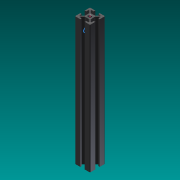
# Autodesk Inventor part: NFS5-2020-170-TPW
Saved by Autodesk Inventor 2015 (Build 190159000, 159)
## iProperties
Category: PARTsolutions
Company: MISUMI
Created: 2016-02-17
Part Number: NFS5-2020-170-TPW
Catalog Web Link: www.cadenas.de
Description: NFS5-2020, NFSB5-2020, HFS5-2020, HFSB5-2020, CAF5-2020, HFSY5-2020, NFSF5-2020, HFSF5-2020, HFSFB5-2020, NFST5-2020, HFST5-2020, HFSTB5-2020, HFSH5-2020, HFSC5-2020-HFS5 Series Aluminum Extrusions 20 Square -1 Slot-
Vendor: MISUMI
Document SubType Name: Modeling
Designer: psAdmin
Manufacturer: MISUMI
Mass: 30.8251 g
Surface Area: 299.433 cm^2
Volume: 30.8251 cm^3
Density: 1 g/cm^3
Material: 一般
Appearance: PSOLRGB-175-175-175
PSOL_IDENT_0: {$CADENAS_DATA\23d-libs\misumi\metric\38_al_extrusions_blackets\5\hfs5_2020.prj},577 {VTYP=3D},{NB=N
PSOL_IDENT_1: FS5-2020-170-TPW},{LINA=NFS5-2020-170-TPW},{NN=NFS5-2020, NFSB5-2020, HFS5-2020, HFSB5-2020, CAF5-20
PSOL_IDENT_2: 20, HFSY5-2020, NFSF5-2020, HFSF5-2020, HFSFB5-2020, NFST5-2020, HFST5-2020, HFSTB5-2020, HFSH5-2020
PSOL_IDENT_3: , HFSC5-2020},{DATE=17.07.2015 10:47:07},{GEOMDATE=28.10.2014 00:00:00},{VERSION=},{LINEID=10},{LINE
PSOL_IDENT_4: SUBID=-1},{WBVAR=L,ALT1,ALT2,ALT4,ALT5,CP5,DL5,DR5,ALT6,ALT9,ALT10,ALT11,HP6,NHL6,DL6,NHR6,DR6,ALT7,
PSOL_IDENT_5: ALT8,NH9,AH,BH,CH,DH,EH,NH10,AV,BV,CV,DV,EV,NH11,AP,BP,CP,DP,EP,ALT12,ALT13,Z,NH12,XA,XB,XC,XD,XE,NH
PSOL_IDENT_6: 13,YA,YB,YC,YD,YE,ALT16,HP16,DL16,DR16,ALT17,HQ17,JLP,ALT20}  {NB=NFS5-2020-170-TPW},{LINA=NFS5-2020
PSOL_IDENT_7: -170-TPW},{KT=DUMMY},{PN=NFS5-2020-170-TPW},{TPS=NFS5-2020},{MAT=6063-T5 Aluminum Alloy},{ST=Clear A
PSOL_IDENT_8: nodize},{FRMW=20},{FRMH=20},{FRD=4.2},{L=170},{MASS=0.5},{SA=183},{LX=0.742x10^4},{LY=0.742x10^4},{A
PSOL_IDENT_9: LT1=TPW},{M1=5},{DPL1=15},{DPR1=15},{ALT1PN=-TPW},{ALT2=},{ALT2ALG= '','Not applicable' },{M2=0},{DP
PSOL_IDENT_10: 2=0},{ALT2PN=},{ALT4=},{ALT4ALG= '', 'w/o SC (High Precision Cut)', 'SC', 'with SC (High Precision C
PSOL_IDENT_11: ut)' },{ALT4PN=},{ALT5=},{ALT5ALG= '','w/o 45 Degree Cut','1','with 45 Degree Cut' },{CP5=},{CP5ALG=
PSOL_IDENT_12: '','N/A' },{DL5=},{DL5ALG= '','N/A' },{DR5=},{DR5ALG= '','N/A' },{FRMLALT5=0},{FRMRALT5=0},{ALT5PN=
PSOL_IDENT_13: },{ALT6=},{ALT6ALG= '','w/o Fastening Location Wrench Access Hole Alterations','1','with Fastening L
PSOL_IDENT_14: ocation Wrench Access Hole Alterations' },{ALT9=},{ALT9ALG= '','w/o Location Specified Wrench Access
PSOL_IDENT_15: Hole Alteratons (Horizontal)','1','with Location Specified Wrench Access Hole Alteratons (Horizonta
PSOL_IDENT_16: l)' },{ALT10=},{ALT10ALG= '','w/o Location Specified Wrench Access Hole Alteratons (Vertical)','1','
PSOL_IDENT_17: with Location Specified Wrench Access Hole Alteratons (Vertical)' },{ALT11=},{ALT11ALG= '','w/o Loca
PSOL_IDENT_18: tion Specified Wrench Access Hole Alteratons (Crisscross)','1','with Location Specified Wrench Acces
PSOL_IDENT_19: s Hole Alteratons (Crisscross)' },{HP6=},{HP6ALG= '','N/A' },{NHL6=},{NHL6ALG= '','N/A' },{DL6=},{DL
PSOL_IDENT_20: 6ALG= '','N/A' },{NHR6=},{NHR6ALG= '','N/A' },{DR6=},{DR6ALG= '','N/A' },{HL6=0},{HL6D=0},{HR6=0},{H
PSOL_IDENT_21: R6D=0},{J6=0},{J6D=0},{K6=0},{K6D=0},{DD6=0.00},{DD6ALG=0},{ALT7=},{ALT7ALG= '','N/A' },{ALT8=},{ALT
PSOL_IDENT_22: 8ALG= '','N/A' },{ALT678PN=},{NH9=0},{NH9MAX=5},{NH9ALG=[0]},{AH=0.0},{AHMIN=7},{AHMAX=165},{AHALG=[
PSOL_IDENT_23: 0]},{BH=0.0},{BHMIN=2},{BHMAX=167},{BHALG=[0]},{CH=0.0},{CHMIN=2},{CHMAX=169},{CHALG=[0]},{DH=0.0},{
PSOL_IDENT_24: DHMIN=2},{DHMAX=171},{DHALG=[0]},{EH=0.0},{EHMIN=2},{EHMAX=163},{EHALG=[0]},{NH10=0},{NH10MAX=5},{NH
PSOL_IDENT_25: 10ALG=[0]},{AV=0.0},{AVMIN=7},{AVMAX=165},{AVALG=[0]},{BV=0.0},{BVMIN=2},{BVMAX=167},{BVALG=[0]},{CV=
PSOL_IDENT_26: 0.0},{CVMIN=2},{CVMAX=169},{CVALG=[0]},{DV=0.0},{DVMIN=2},{DVMAX=171},{DVALG=[0]},{EV=0.0},{EVMIN=2}
PSOL_IDENT_27: ,{EVMAX=163},{EVALG=[0]},{NH11=0},{NH11MAX=5},{NH11ALG=[0]},{AP=0.0},{APMIN=7},{APMAX=165},{APALG=[0
PSOL_IDENT_28: ]},{BP=0.0},{BPMIN=2},{BPMAX=167},{BPALG=[0]},{CP=0.0},{CPMIN=2},{CPMAX=169},{CPALG=[0]},{DP=0.0},{D
PSOL_IDENT_29: PMIN=2},{DPMAX=171},{DPALG=[0]},{EP=0.0},{EPMIN=2},{EPMAX=163},{EPALG=[0]},{ALT9PN=},{ALT10PN=},{ALT
PSOL_IDENT_30: 11PN=},{ALT91011PN=},{ALT12=},{ALT12ALG= '','w/o Counterbore Hole in Specified Position (Vertical)','
PSOL_IDENT_31: 1','with Counterbore Hole in Specified Position (Vertical)' },{ALT13=},{ALT13ALG= '','w/o Counterbor
PSOL_IDENT_32: e Hole in Specified Position (Horizontal)','1','with Counterbore Hole in Specified Position (Horizon
PSOL_IDENT_33: tal)' },{Z=},{ZALG= '','N/A' },{DD12=0.0},{DD112=0.0},{NH12=0},{NH12MAX=5},{NH12ALG=[0]},{XA=0.0},{X
PSOL_IDENT_34: AMIN=7},{XAMAX=165},{XAALG=[0]},{XB=0.0},{XBMIN=2},{XBMAX=167},{XBALG=[0]},{XC=0.0},{XCMIN=2},{XCMAX=
PSOL_IDENT_35: 169},{XCALG=[0]},{XD=0.0},{XDMIN=2},{XDMAX=171},{XDALG=[0]},{XE=0.0},{XEMIN=2},{XEMAX=163},{XEALG=[0
PSOL_IDENT_36: ]},{NH13=0},{NH13MAX=5},{NH13ALG=[0]},{YA=0.0},{YAMIN=7},{YAMAX=165},{YAALG=[0]},{YB=0.0},{YBMIN=2},
PSOL_IDENT_37: {YBMAX=167},{YBALG=[0]},{YC=0.0},{YCMIN=2},{YCMAX=169},{YCALG=[0]},{YD=0.0},{YDMIN=2},{YDMAX=171},{Y
PSOL_IDENT_38: DALG=[0]},{YE=0.0},{YEMIN=2},{YEMAX=163},{YEALG=[0]},{ALT12PN=},{ALT13PN=},{ALT1213PN=},{ALT16=},{AL
PSOL_IDENT_39: T16ALG= '','w/o M Type Hole Alteration','1','with M Type Hole Alteration' },{HP16=},{HP16ALG= '','N/
PSOL_IDENT_40: A' },{DL16=},{DL16ALG= '','N/A' },{DR16=},{DR16ALG= '','N/A' },{H116=0},{D16=0.0},{ALT16PN=},{ALT17=
PSOL_IDENT_41: },{ALT17ALG= '','w/o L Type Hole Alteration (Top)','1','with L Type Hole Alteration (Top)' },{HQ17=0
PSOL_IDENT_42: },{HQ17ALG=0},{JLP=0},{JLPMIN=4.9},{JLPMAX=0},{JLPALG=[0]},{L17=0},{D17=0.0},{ALT17PN=},{ALT20=},{AL
PSOL_IDENT_43: T20PN=},{ERRORALT01=OK},{ERRORALT02=OK},{ERRORALT05=OK},{ERRORALT06091=OK},{ERRORALT06092=OK},{ERROR
PSOL_IDENT_44: ALT06093=OK},{ERRORALT06094=OK},{ERRORALT06101=OK},{ERRORALT06102=OK},{ERRORALT06103=OK},{ERRORALT06
PSOL_IDENT_45: 104=OK},{ERRORALT06111=OK},{ERRORALT06112=OK},{ERRORALT06113=OK},{ERRORALT06114=OK},{ERRORALT06121=O
PSOL_IDENT_46: K},{ERRORALT06122=OK},{ERRORALT06123=OK},{ERRORALT06124=OK},{ERRORALT06131=OK},{ERRORALT06132=OK},{E
PSOL_IDENT_47: RRORALT06133=OK},{ERRORALT06134=OK},{ERRORALT0616=OK},{ERRORALT06171=OK},{ERRORALT06172=OK},{ERRORAL
PSOL_IDENT_48: T06173=OK},{ERRORALT0911=OK},{ERRORALT0913=OK},{ERRORALT0916=OK},{ERRORALT0917=OK},{ERRORALT1011=OK}
PSOL_IDENT_49: ,{ERRORALT1012=OK},{ERRORALT1016=OK},{ERRORALT1017=OK},{ERRORALT1112=OK},{ERRORALT1113=OK},{ERRORALT
PSOL_IDENT_50: 1116=OK},{ERRORALT1117=OK},{ERRORALT1216=OK},{ERRORALT1217=OK},{ERRORALT1316=OK},{ERRORALT1317=OK},{
PSOL_IDENT_51: ERRORALT1617=OK},{ERRORPN=},{TFW=0}
NN: NFS5-2020, NFSB5-2020, HFS5-2020, HFSB5-2020, CAF5-2020, HFSY5-2020, NFSF5-2020, HFSF5-2020, HFSFB5-2020, NFST5-2020, HFST5-2020, HFSTB5-2020, HFSH5-2020, HFSC5-2020
NT: HFS5 Series Aluminum Extrusions 20 Square -1 Slot-
NB: NFS5-2020-170-TPW
NBSYN: $PN.
LINA: NFS5-2020-170-TPW
PN: NFS5-2020-170-TPW
TPS: NFS5-2020
MAT: 6063-T5 Aluminum Alloy
ST: Clear Anodize
L: 170
MASS: 0.5
SA: 183
LX: 0.742x10^4
LY: 0.742x10^4
ALT1: with TPW (Tapping on Both Ends)
M1: 5
DPL1: 15
DPR1: 15
ALT2: Not applicable
M2: 0
DP2: 0
ALT4: w/o SC (High Precision Cut)
ALT5: w/o 45 Degree Cut
CP5: N/A
DL5: N/A
DR5: N/A
ALT6: w/o Fastening Location Wrench Access Hole Alterations
ALT9: w/o Location Specified Wrench Access Hole Alteratons (Horizontal)
ALT10: w/o Location Specified Wrench Access Hole Alteratons (Vertical)
ALT11: w/o Location Specified Wrench Access Hole Alteratons (Crisscross)
HP6: N/A
NHL6: N/A
DL6: N/A
NHR6: N/A
DR6: N/A
HL6D: 0
HR6D: 0
J6D: 0
K6D: 0
DD6: 0.00
ALT7: N/A
ALT8: N/A
NH9: 0
AH: 0.0
BH: 0.0
CH: 0.0
DH: 0.0
EH: 0.0
NH10: 0
AV: 0.0
BV: 0.0
CV: 0.0
DV: 0.0
EV: 0.0
NH11: 0
AP: 0.0
BP: 0.0
CP: 0.0
DP: 0.0
EP: 0.0
ALT12: w/o Counterbore Hole in Specified Position (Vertical)
ALT13: w/o Counterbore Hole in Specified Position (Horizontal)
Z: N/A
DD12: 0.0
DD112: 0.0
NH12: 0
XA: 0.0
XB: 0.0
XC: 0.0
XD: 0.0
XE: 0.0
NH13: 0
YA: 0.0
YB: 0.0
YC: 0.0
YD: 0.0
YE: 0.0
ALT16: w/o M Type Hole Alteration
HP16: N/A
DL16: N/A
DR16: N/A
H116: 0
D16: 0.0
ALT17: w/o L Type Hole Alteration (Top)
HQ17: 0
JLP: 0
D17: 0.0
ALT20: w/o CW (End Face C Chamfering)
SUPPLIER: MISUMI
ARTICLENO: NFS5-2020-170-TPW
BOMINFO: NFS5-2020-170-TPW
CREATOR: CADENAS GmbH
Title: NFS5-2020-170-TPW
Author: Cadenas PARTsolutions
Comments: HFS5 Series Aluminum Extrusions 20 Square -1 Slot-
Autodesk Inventor part; units mm, degrees
sketch "Sketch_75" plane through (0, 0, 0) normal (0, 0, 1) x (1, 0, 0)
  line L0 (-10, 3) -> (-8, 3)
  line L1 (-8, 3) -> (-8, 6)
  line L2 (-8, 6) -> (-7.0607, 6)
  line L3 (-7.0607, 6) -> (-4, 2.9393)
  line L4 (-4, 2.9393) -> (-4, 0.6536)
  arc A0 (-4, 0.6536) -> (-3.933, 0.4036) centre (-3.5, 0.6536) ccw
  line L5 (-3.933, 0.4036) -> (-3.7, 0)
  line L6 (-3.7, 0) -> (-3.933, -0.4036)
  arc A1 (-3.933, -0.4036) -> (-3.933, -0.9036) centre (-3.5, -0.6536) ccw
  line L7 (-3.933, -0.9036) -> (-3.751, -1.2189)
  line L8 (-3.751, -1.2189) -> (-4, -2.5)
  line L9 (-4, -2.5) -> (-4, -2.9393)
  line L10 (-4, -2.9393) -> (-7.0607, -6)
  line L11 (-7.0607, -6) -> (-8, -6)
  line L12 (-8, -6) -> (-8, -3)
  line L13 (-8, -3) -> (-10, -3)
  line L14 (-10, -3) -> (-10, -9)
  arc A2 (-10, -9) -> (-9, -10) centre (-9, -9) ccw
  line L15 (-9, -10) -> (-3, -10)
  line L16 (-3, -10) -> (-3, -8)
  line L17 (-3, -8) -> (-6, -8)
  line L18 (-6, -8) -> (-6, -7.0607)
  line L19 (-6, -7.0607) -> (-2.9393, -4)
  line L20 (-2.9393, -4) -> (-0.6536, -4)
  arc A3 (-0.6536, -4) -> (-0.4036, -3.933) centre (-0.6536, -3.5) ccw
  line L21 (-0.4036, -3.933) -> (0, -3.7)
  line L22 (0, -3.7) -> (0.4036, -3.933)
  arc A4 (0.4036, -3.933) -> (0.9036, -3.933) centre (0.6536, -3.5) ccw
  line L23 (0.9036, -3.933) -> (1.2189, -3.751)
  line L24 (1.2189, -3.751) -> (2.5, -4)
  line L25 (2.5, -4) -> (2.9393, -4)
  line L26 (2.9393, -4) -> (6, -7.0607)
  line L27 (6, -7.0607) -> (6, -8)
  line L28 (6, -8) -> (3, -8)
  line L29 (3, -8) -> (3, -10)
  line L30 (3, -10) -> (9, -10)
  arc A5 (9, -10) -> (10, -9) centre (9, -9) ccw
  line L31 (10, -9) -> (10, -3)
  line L32 (10, -3) -> (8, -3)
  line L33 (8, -3) -> (8, -6)
  line L34 (8, -6) -> (7.0607, -6)
  line L35 (7.0607, -6) -> (4, -2.9393)
  line L36 (4, -2.9393) -> (4, -0.6536)
  arc A6 (4, -0.6536) -> (3.933, -0.4036) centre (3.5, -0.6536) ccw
  line L37 (3.933, -0.4036) -> (3.7, 0)
  line L38 (3.7, 0) -> (3.933, 0.4036)
  arc A7 (3.933, 0.4036) -> (3.933, 0.9036) centre (3.5, 0.6536) ccw
  line L39 (3.933, 0.9036) -> (3.751, 1.2189)
  line L40 (3.751, 1.2189) -> (4, 2.5)
  line L41 (4, 2.5) -> (4, 2.9393)
  line L42 (4, 2.9393) -> (7.0607, 6)
  line L43 (7.0607, 6) -> (8, 6)
  line L44 (8, 6) -> (8, 3)
  line L45 (8, 3) -> (10, 3)
  line L46 (10, 3) -> (10, 9)
  arc A8 (10, 9) -> (9, 10) centre (9, 9) ccw
  line L47 (9, 10) -> (3, 10)
  line L48 (3, 10) -> (3, 8)
  line L49 (3, 8) -> (6, 8)
  line L50 (6, 8) -> (6, 7.0607)
  line L51 (6, 7.0607) -> (2.9393, 4)
  line L52 (2.9393, 4) -> (0.6536, 4)
  arc A9 (0.6536, 4) -> (0.4036, 3.933) centre (0.6536, 3.5) ccw
  line L53 (0.4036, 3.933) -> (0, 3.7)
  line L54 (0, 3.7) -> (-0.4036, 3.933)
  arc A10 (-0.4036, 3.933) -> (-0.9036, 3.933) centre (-0.6536, 3.5) ccw
  line L55 (-0.9036, 3.933) -> (-1.2189, 3.751)
  line L56 (-1.2189, 3.751) -> (-2.5, 4)
  line L57 (-2.5, 4) -> (-2.9393, 4)
  line L58 (-2.9393, 4) -> (-6, 7.0607)
  line L59 (-6, 7.0607) -> (-6, 8)
  line L60 (-6, 8) -> (-3, 8)
  line L61 (-3, 8) -> (-3, 10)
  line L62 (-3, 10) -> (-9, 10)
  arc A11 (-9, 10) -> (-10, 9) centre (-9, 9) ccw
  line L63 (-10, 9) -> (-10, 3)
  constraints: 128 end point, 24 point on circle, 12 centre point
extrude "Extrusion1" add sketch "Sketch_75" against normal blind 170
sketch "Sketch2" plane through (0, 0, 0) normal (0, 0, 1) x (1, 0, 0)
  point P0 (0, 0)
hole "Hole1" at (0, 0, 0) direction (0, 0, -1) diameter 4.134 depth 15 countersink diameter 5 countersink angle 90 thread size "M5x0.8" class "6H" standard "ISO Metric profile"
sketch "Sketch3" plane through (0, 0, -170) normal (0, 0, -1) x (-1, 0, 0)
  point P0 (0, 0)
hole "Hole2" at (0, 0, -170) direction (0, 0, 1) diameter 4.134 depth 15 countersink diameter 5 countersink angle 90 thread size "M5x0.8" class "6H" standard "ISO Metric profile"
sketch "Sketch4" plane through (0, 0, -155) normal (0, 0, -1) x (-1, 0, 0)
  point P0 (0, 0)
hole "Hole3" at (0, 0, -155) direction (0, 0, 1) diameter 4.2 depth 140
ref_plane "C1_XY" through (0, 0, 0) normal (0, 0, 1) x (1, 0, 0)
ref_plane "C1_YZ" through (0, 0, 0) normal (1, 0, 0) x (0, 1, 0)
ref_plane "C1_ZX" through (0, 0, 0) normal (0, 1, 0) x (0, 0, 1)
sketch "スケッチ5" plane through (0, 0, 0) normal (1, 0, 0) x (0, 1, 0)
  circle A0 centre (0.6157, -9.9012) radius 2.5558
  circle A1 centre (-5.1594, -12.6083) radius 3.4704
  point P0 (0, 0)
  point P1 (0.6157, -9.42)
  point P2 (0.6157, -10.3223)
  point P3 (0.6157, -11.0442)
  point P4 (0.6157, -11.0442)
  constraints: 2 centre point, 1 coincident
sketch "スケッチ6" plane through (10, 3, 0) normal (1, 0, 0) x (0, 0, -1)
  line L0 (0, -12) -> (0, -6) projected
  line L1 (0, -13) -> (170, -13) projected
  point P0 (0, -3)
  point P1 (10, -3)
  dimension "d24" = 10
  dimension "d32" = 10
  measures "d24" distance from line of L0 point (10, -3)
  measures "d32" distance from line of L1 point (10, -3)
hole "穴4" at (10, 0, -10) direction (-1, 0, 0) diameter 5.5 end through all
body "Solid1"
